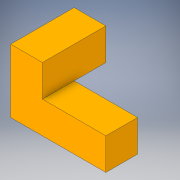
# Autodesk Inventor part: OrangePiece
Saved by Autodesk Inventor 2019 (Build 230136000, 136)
## iProperties
Created: 2018-12-10
Part Number: OrangePiece
Material: Generic
Document SubType Name: Modeling
Designer: Mihir
Density: 1 g/cm^3
Appearance: Default
Author: Mihir
Autodesk Inventor part; units mm, degrees
ref_plane "YZ Plane" through (0, 0, 0) normal (1, 0, 0) x (0, 1, 0)
ref_plane "XZ Plane" through (0, 0, 0) normal (0, 1, 0) x (-1, 0, 0)
ref_plane "XY Plane" through (0, 0, 0) normal (0, 0, 1) x (1, 0, 0)
sketch "Sketch3" plane through (0, 0, 0) normal (0, 0, 1) x (1, 0, 0)
  line L0 (0, 0) -> (57.15, 0)
  line L1 (57.15, 0) -> (57.15, 19.05)
  line L2 (57.15, 19.05) -> (0, 19.05)
  line L3 (0, 19.05) -> (0, 0)
  line L4 (0, 19.05) -> (19.05, 19.05)
  line L5 (19.05, 19.05) -> (19.05, 38.1)
  line L6 (19.05, 38.1) -> (0, 38.1)
  line L7 (0, 38.1) -> (0, 19.05)
  dimension "d9" = 57.15
  dimension "d10" = 19.05
  dimension "d11" = 19.05
  dimension "d12" = 19.05
  constraints: 16 end point, 4 parallel, 2 horizontal, 2 perpendicular
  measures "d9" distance of L1.end L2.end
  measures "d10" distance of L0.end L1.end
  measures "d11" distance of L5.end L6.end
  measures "d12" distance of L6.end L2.end
extrude "Extrusion3" add sketch "Sketch3" along normal blind 19.05
sketch "Sketch4" plane through (0, 0, 0) normal (0, 0, -1) x (-1, 0, 0)
  line L0 (-19.05, 19.05) -> (-19.05, 38.1) projected
  line L1 (-19.05, 38.1) -> (0, 38.1) projected
  line L2 (-19.05, 19.05) -> (0, 19.05)
  line L3 (0, 19.05) -> (0, 38.1)
  line L4 (0, 38.1) -> (-19.05, 38.1)
  line L5 (-19.05, 38.1) -> (-19.05, 19.05)
  point P0 (0, 0)
  constraints: 8 end point, 2 parallel, 1 horizontal, 1 perpendicular
extrude "Extrusion4" add sketch "Sketch4" along normal blind 19.05
body "Solid2"
